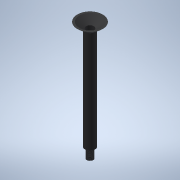
# Autodesk Inventor part: Fuss1,0
Saved by Autodesk Inventor 2021.3 (Build 253353000, 353)
## iProperties
Created: 2021-10-11
Part Number: Fuss1,0
Material: Generisch
Document SubType Name: Modeling
Designer: bhelg
Density: 1 g/cm^3
Appearance: Generisch
Author: bhelg
Autodesk Inventor part; units mm, degrees
ref_plane "YZ Plane" through (0, 0, 0) normal (1, 0, 0) x (0, 1, 0)
ref_plane "XZ Plane" through (0, 0, 0) normal (0, 1, 0) x (-1, 0, 0)
ref_plane "XY Plane" through (0, 0, 0) normal (0, 0, 1) x (1, 0, 0)
sketch "Skizze1" plane through (0, 0, 0) normal (1, 0, 0) x (0, 1, 0)
  line L0 (0, 0) -> (2.5, 0)
  line L1 (0, 0) -> (2.5, 0) construction
  line L2 (2.5, 0) -> (2.5, 7)
  line L3 (2.5, 7) -> (2, 7.5)
  line L4 (2, 7.5) -> (2, 8)
  line L5 (2, 8) -> (4, 8)
  line L6 (4, 8) -> (4, 88)
  line L7 (0, 93) -> (9.9588, 93)
  line L8 (9.9588, 93) -> (4, 88)
  line L9 (0, 0) -> (0, 93)
  line L10 (0, -18.6) -> (0, 111.6) projected
  dimension "d0" = 2.5
  dimension "d1" = 0
  dimension "d2" = 7
  dimension "d4" = 0.5
  dimension "d5" = 0.5
  dimension "d6" = 2
  dimension "d7" = 4
  dimension "d23" = 40
  dimension "d24" = 5
  dimension "d25" = 85
  constraints: 20 end point, 4 horizontal, 3 perpendicular, 2 parallel, 1 collinear
  measures "d0" distance of L0.start L0.end
  measures "d1" distance between parallel lines of L0 L1
  measures "d2" distance of L0.end L2.end
  measures "d4" distance of L3.end L4.end
  measures "d5" horizontal distance of L2.end L3.end
  measures "d6" distance from line of L4 L0.start
  measures "d7" distance from line of L0.start L6
  measures "d23" angle of L8 L7
  measures "d24" vertical distance of L7.end L6.end
  measures "d25" distance between parallel lines of L7 L5
revolve "Umdrehung1" add sketch "Skizze1" angle 360 about axis through (0, 0, -10) along (0, 0, 1)
thread "Gewinde1" size "M5x0.8" class "6g" standard "ANSI Metric M Profile" full length
shell "Wandung4" thickness 1 removed faces 1 at (-0.1358, 2.201, 93)
